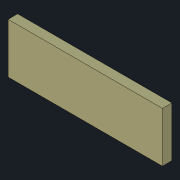
# Autodesk Inventor part: Table
Saved by Autodesk Inventor 2022 (Build 260153000, 153)
## iProperties
Created: 2021-12-06
Part Number: Table
Material: Generic
Document SubType Name: Modeling
Designer: alber
Density: 1 g/cm^3
Appearance: Default
Author: alber
Autodesk Inventor part; units mm, degrees
ref_plane "YZ Plane" through (0, 0, 0) normal (1, 0, 0) x (0, 1, 0)
ref_plane "XZ Plane" through (0, 0, 0) normal (0, 1, 0) x (-1, 0, 0)
ref_plane "XY Plane" through (0, 0, 0) normal (0, 0, 1) x (1, 0, 0)
sketch "Sketch1" plane through (0, 0, 0) normal (0, 0, 1) x (1, 0, 0)
  line L0 (-198.4602, 0) -> (214.3004, 0)
  line L1 (214.3004, 0) -> (214.3004, 118.9542)
  line L2 (214.3004, 118.9542) -> (-198.4602, 118.9542)
  line L3 (-198.4602, 118.9542) -> (-198.4602, 0)
  point P0 (0, 0)
  constraints: 8 end point, 2 parallel, 1 horizontal, 1 perpendicular
extrude "Extrusion1" add sketch "Sketch1" along normal blind 25.4
move faces "Move1" translate (0, -14.8951, 0) faces at (-60.8733, 0, 8.4667)
move faces "Move2" translate (0, 107.95, 0) faces at (-60.8733, 118.9542, 16.9333)
move faces "Move3" translate (-122.2502, 0, 0) faces at (-198.4602, 65.7047, 16.9333)
move faces "Move4" translate (98.425, 0, 0) faces at (-320.7104, 65.7047, 16.9333)
body "Solid1"
